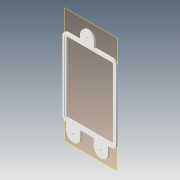
# Autodesk Inventor part: Omniscope_Wellcarrier
Saved by Autodesk Inventor 2022 (Build 260153000, 153)
## iProperties
Created: 2022-05-31
Part Number: Omniscope_Wellcarrier
Material: Generisch
Document SubType Name: Modeling
Designer: diederichbenedict
Density: 1 g/cm^3
Appearance: Vorgabe
Author: diederichbenedict
Autodesk Inventor part; units mm, degrees
ref_plane "YZ Plane" through (0, 0, 0) normal (1, 0, 0) x (0, 1, 0)
ref_plane "XZ Plane" through (0, 0, 0) normal (0, 1, 0) x (-1, 0, 0)
ref_plane "XY Plane" through (0, 0, 0) normal (0, 0, 1) x (1, 0, 0)
ref_plane "Arbeitsebene1" through (0, 0, 0) normal (0, 0, 1) x (1, 0, 0)
sketch "Skizze1" plane through (0, 0, 0) normal (0, 0, 1) x (1, 0, 0)
  line L0 (-42.8, 60.945) -> (-42.8, -60.945) construction
  arc A0 (-42.8, -60.945) -> (-39.8, -63.945) centre (-39.8, -60.945) ccw construction
  line L1 (-39.8, -63.945) -> (39.8, -63.945) construction
  arc A1 (39.8, -63.945) -> (42.8, -60.945) centre (39.8, -60.945) ccw construction
  line L2 (42.8, -60.945) -> (42.8, 60.945) construction
  arc A2 (42.8, 60.945) -> (39.8, 63.945) centre (39.8, 60.945) ccw construction
  line L3 (39.8, 63.945) -> (-39.8, 63.945) construction
  arc A3 (-39.8, 63.945) -> (-42.8, 60.945) centre (-39.8, 60.945) ccw construction
  line L4 (-41.3, 51.2024) -> (-41.3, -59.445) construction
  arc A4 (-40.4213, 53.3237) -> (-41.3, 51.2024) centre (-38.3, 51.2024) ccw construction
  line L5 (-40.4213, 53.3237) -> (-32.1787, 61.5663) construction
  arc A5 (-30.0574, 62.445) -> (-32.1787, 61.5663) centre (-30.0574, 59.445) ccw construction
  line L6 (30.0574, 62.445) -> (-30.0574, 62.445) construction
  arc A6 (32.1787, 61.5663) -> (30.0574, 62.445) centre (30.0574, 59.445) ccw construction
  line L7 (32.1787, 61.5663) -> (40.4213, 53.3237) construction
  arc A7 (41.3, 51.2024) -> (40.4213, 53.3237) centre (38.3, 51.2024) ccw construction
  line L8 (41.3, -59.445) -> (41.3, 51.2024) construction
  arc A8 (38.3, -62.445) -> (41.3, -59.445) centre (38.3, -59.445) ccw construction
  line L9 (-38.3, -62.445) -> (38.3, -62.445) construction
  arc A9 (-41.3, -59.445) -> (-38.3, -62.445) centre (-38.3, -59.445) ccw construction
  line L10 (41.3, 60.945) -> (41.3, -60.945)
  arc A10 (39.8, -62.445) -> (41.3, -60.945) centre (39.8, -60.945) ccw
  line L11 (39.8, -62.445) -> (-39.8, -62.445)
  arc A11 (-41.3, -60.945) -> (-39.8, -62.445) centre (-39.8, -60.945) ccw
  line L12 (-41.3, -60.945) -> (-41.3, 60.945)
  arc A12 (-39.8, 62.445) -> (-41.3, 60.945) centre (-39.8, 60.945) ccw
  line L13 (-39.8, 62.445) -> (39.8, 62.445)
  arc A13 (41.3, 60.945) -> (39.8, 62.445) centre (39.8, 60.945) ccw
  line L14 (47.8, 60.945) -> (47.8, -60.945)
  arc A14 (39.8, -68.945) -> (47.8, -60.945) centre (39.8, -60.945) ccw
  line L15 (39.8, -68.945) -> (-39.8, -68.945)
  arc A15 (-47.8, -60.945) -> (-39.8, -68.945) centre (-39.8, -60.945) ccw
  line L16 (-47.8, -60.945) -> (-47.8, 60.945)
  arc A16 (-39.8, 68.945) -> (-47.8, 60.945) centre (-39.8, 60.945) ccw
  line L17 (-39.8, 68.945) -> (39.8, 68.945)
  arc A17 (47.8, 60.945) -> (39.8, 68.945) centre (39.8, 60.945) ccw
  circle A18 centre (-3.75, 78.25) radius 8.5 projected
  circle A19 centre (20.75, -81.65) radius 8.5 projected
  circle A20 centre (-28.25, -81.65) radius 8.5 projected
  circle A21 centre (20.75, -81.65) radius 12.705
  circle A22 centre (-28.25, -81.65) radius 12.705
  circle A23 centre (-3.75, 78.25) radius 12.5
  line L18 (8.75, 78.25) -> (8.75, 68.945)
  line L19 (-16.25, 78.25) -> (-16.25, 68.945)
  line L20 (-40.955, -81.65) -> (-40.955, -68.8612)
  line L21 (-15.545, -81.65) -> (-15.545, -68.945)
  line L22 (8.045, -81.65) -> (8.045, -68.945)
  line L23 (33.455, -81.65) -> (33.455, -68.945)
  circle A24 centre (-3.75, 78.25) radius 1.4
  circle A25 centre (20.75, -81.65) radius 1.4
  circle A26 centre (-28.25, -81.65) radius 1.4
  point P0 (0, 0)
  dimension "d0" = 5
  dimension "d1" = 1.5
  dimension "d2" = 25
  dimension "d3" = 2.8
  dimension "d4" = 2.8
  dimension "d5" = 2.8
  constraints: 28 end point, 23 point on circle, 14 centre point, 8 tangent, 6 coincident, 5 perpendicular, 5 point on line, 1 parallel, 14 other
  measures "d0" distance between parallel lines of L2 L14
  measures "d1" distance between parallel lines of L10 L2
  measures "d2" diameter of A23
  measures "d3" diameter of A24
  measures "d4" diameter of A25
  measures "d5" diameter of A26
extrude "Extrusion1" add sketch "Skizze1" along normal blind 3 contours L14 A14 L15 A15 L16 A16 L17 A23 A17 | L17 A23 L18 | L23 A21 L15 | A23 L17 | L17 A23 | A21 L22 L15 | A21 | L17 L19 A23 | L21 A22 L15 | A22 L20 A15 L15 | A22 | A18 | A19 | A20
sketch "Skizze2" plane through (0, 0, 3) normal (0, 0, 1) x (1, 0, 0)
  line L0 (-42.8, 60.945) -> (-42.8, -60.945) projected
  arc A0 (-42.8, -60.945) -> (-39.8, -63.945) centre (-39.8, -60.945) ccw projected
  line L1 (-39.8, -63.945) -> (39.8, -63.945) projected
  arc A1 (39.8, -63.945) -> (42.8, -60.945) centre (39.8, -60.945) ccw projected
  line L2 (42.8, -60.945) -> (42.8, 60.945) projected
  arc A2 (42.8, 60.945) -> (39.8, 63.945) centre (39.8, 60.945) ccw projected
  line L3 (39.8, 63.945) -> (-39.8, 63.945) projected
  arc A3 (-39.8, 63.945) -> (-42.8, 60.945) centre (-39.8, 60.945) ccw projected
  line L4 (-41.3, 51.2024) -> (-41.3, -59.445) projected
  arc A4 (-40.4213, 53.3237) -> (-41.3, 51.2024) centre (-38.3, 51.2024) ccw projected
  line L5 (-40.4213, 53.3237) -> (-32.1787, 61.5663) projected
  arc A5 (-30.0574, 62.445) -> (-32.1787, 61.5663) centre (-30.0574, 59.445) ccw projected
  line L6 (30.0574, 62.445) -> (-30.0574, 62.445) projected
  arc A6 (32.1787, 61.5663) -> (30.0574, 62.445) centre (30.0574, 59.445) ccw projected
  line L7 (32.1787, 61.5663) -> (40.4213, 53.3237) projected
  arc A7 (41.3, 51.2024) -> (40.4213, 53.3237) centre (38.3, 51.2024) ccw projected
  line L8 (41.3, -59.445) -> (41.3, 51.2024) projected
  arc A8 (38.3, -62.445) -> (41.3, -59.445) centre (38.3, -59.445) ccw projected
  line L9 (-38.3, -62.445) -> (38.3, -62.445) projected
  arc A9 (-41.3, -59.445) -> (-38.3, -62.445) centre (-38.3, -59.445) ccw projected
  line L10 (43.8, 60.945) -> (43.8, -60.945)
  arc A10 (39.8, -64.945) -> (43.8, -60.945) centre (39.8, -60.945) ccw
  line L11 (39.8, -64.945) -> (-39.8, -64.945)
  arc A11 (-43.8, -60.945) -> (-39.8, -64.945) centre (-39.8, -60.945) ccw
  line L12 (-43.8, -60.945) -> (-43.8, 60.945)
  arc A12 (-39.8, 64.945) -> (-43.8, 60.945) centre (-39.8, 60.945) ccw
  line L13 (-39.8, 64.945) -> (39.8, 64.945)
  arc A13 (43.8, 60.945) -> (39.8, 64.945) centre (39.8, 60.945) ccw
  point P0 (0, 0)
  dimension "d8" = 1
  constraints: 8 end point, 8 point on circle, 4 centre point, 7 other
  measures "d8" distance between parallel lines of L2 L10
extrude "Extrusion2" cut sketch "Skizze2" against normal blind 1 contours A3 L3 A2 L2 A1 L1 A0 L0 | A4 L5 A5 L6 A6 L7 A7 L8 A8 L9 A9 L4 | L10 A10 L11 A11 L12 A12 L13 A13
